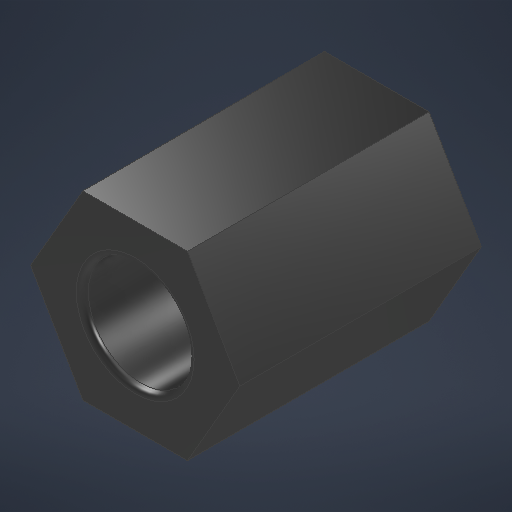
# Autodesk Inventor part: Espaçador_m3_L5
Saved by Autodesk Inventor 2025.2 (Build 292293000, 293)
## iProperties
Created: 2025-05-14
Part Number: Espaçador_m3_L5
Material: PLA Plastic
Document SubType Name: Modeling
Designer: Tiago
Density: 1.18 g/cm^3
Appearance: Generic(1)
Mass: 0.109959 g
Surface Area: 1.84905 cm^2
Volume: 0.0931857 cm^3
Author: Tiago
Autodesk Inventor part; units mm, degrees
ref_plane "YZ Plane" through (0, 0, 0) normal (1, 0, 0) x (0, 1, 0)
ref_plane "XZ Plane" through (0, 0, 0) normal (0, 1, 0) x (-1, 0, 0)
ref_plane "XY Plane" through (0, 0, 0) normal (0, 0, 1) x (1, 0, 0)
sketch "Sketch1" plane through (0, 0, 0) normal (0, 0, 1) x (1, 0, 0)
  circle A0 centre (0, 0) radius 1.75
  circle A1 centre (0, 0) radius 3
  line L0 (1.7321, 3) -> (3.4641, 0)
  line L1 (3.4641, 0) -> (1.7321, -3)
  line L2 (1.7321, -3) -> (-1.7321, -3)
  line L3 (-1.7321, -3) -> (-3.4641, 0)
  line L4 (-3.4641, 0) -> (-1.7321, 3)
  line L5 (-1.7321, 3) -> (1.7321, 3)
  point P0 (0, 3)
  point P1 (0, 3)
  point P2 (-2.5981, 1.5)
  point P3 (2.5981, 1.5)
  point P4 (-2.5981, -1.5)
  point P5 (0, -3)
  point P6 (2.5981, -1.5)
  dimension "Di" = 3.5
  dimension "d1" = 6
  dimension "d5" = 6
  constraints: 12 end point, 3 coincident, 2 centre point, 1 midpoint, 1 vertical alignment, 13 other
  measures "Di" diameter of A0
  measures "d1" diameter of A1
  measures "d5" distance between parallel lines of L2 L5
extrude "Extrusion1" add sketch "Sketch1" along normal blind 8
fillet "Fillet2" radius 0.2 2 edges at (-1.75, 0, 0) (-1.75, 0, 8)
body "Solid1"
